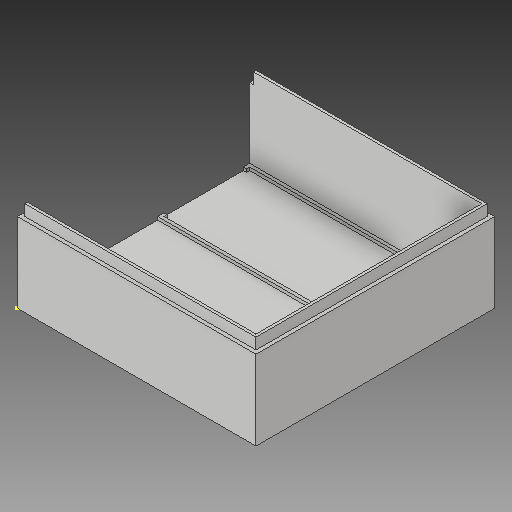
# Autodesk Inventor part: base inf
Saved by Autodesk Inventor 2018.2 (Build 222227000, 227)
## iProperties
Created: 2016-05-12
Part Number: base inf
Material: Genérico
Document SubType Name: Modeling
Designer: Usuario
Density: 1 g/cm^3
Appearance: Valor por defecto
Author: Usuario
Autodesk Inventor part; units mm, degrees
ref_plane "YZ Plane" through (0, 0, 0) normal (1, 0, 0) x (0, 1, 0)
ref_plane "XZ Plane" through (0, 0, 0) normal (0, 1, 0) x (-1, 0, 0)
ref_plane "XY Plane" through (0, 0, 0) normal (0, 0, 1) x (1, 0, 0)
sketch "Boceto1" plane through (0, 0, 0) normal (0, 1, 0) x (-1, 0, 0)
  line L0 (0, 0) -> (0, -150)
  line L1 (0, -150) -> (-150, -150)
  line L2 (-150, -150) -> (-150, 0)
  line L3 (-150, 0) -> (0, 0)
  constraints: 8 end point, 2 perpendicular, 1 vertical
extrude "Extrusión1" add sketch "Boceto1" along normal blind 4
sketch "Boceto2" plane through (0, 4, 0) normal (0, 1, 0) x (1, 0, 0)
  line L0 (0, 150) -> (4, 150)
  line L1 (150, 150) -> (0, 150) projected
  line L2 (0, 150) -> (0, 0)
  line L3 (0, 0) -> (150, 0)
  line L4 (150, 0) -> (150, 150)
  line L5 (0, 150) -> (150, 150)
  line L6 (4, 4) -> (146, 4)
  line L7 (146, 146) -> (146, 4)
  line L8 (146, 146) -> (4, 146)
  line L9 (4, 4) -> (4, 146)
  constraints: 18 end point, 4 perpendicular, 1 horizontal, 1 point on line, 1 vertical
extrude "Extrusión2" add sketch "Boceto2" along normal blind 46
sketch "Boceto3" plane through (0, 0, 0) normal (0, 0, 1) x (1, 0, 0)
  point P0 (0, 0)
sketch "Boceto4" plane through (0, 50, 0) normal (0, 1, 0) x (1, 0, 0)
  line L0 (4, 146) -> (146, 146) projected
  line L1 (0, 0) -> (0, 150) projected
  line L2 (146, 4) -> (4, 4) projected
  line L3 (2.3, 4) -> (2.3, 147.7)
  line L4 (2.3, 4) -> (2.3, 2.3)
  line L5 (2.3, 2.3) -> (147.7, 2.3)
  line L6 (147.7, 147.7) -> (2.3, 147.7)
  line L7 (147.7, 147.7) -> (147.7, 2.3)
  line L8 (4, 146) -> (146, 146)
  line L9 (146, 146) -> (146, 4) projected
  line L10 (146, 4) -> (146, 146)
  line L11 (4, 146) -> (4, 4)
  line L12 (4, 4) -> (146, 4)
  constraints: 18 end point, 5 perpendicular, 1 collinear, 1 parallel, 1 vertical
extrude "Extrusión3" add sketch "Boceto4" along normal blind 7
sketch "Boceto5" plane through (0, 0, -150) normal (-1, 0, 0) x (0, 0, 1)
  point P0 (150, 0)
sketch "Boceto6" plane through (0, 0, -150) normal (-1, 0, 0) x (0, 0, 1)
  line L0 (0, 0) -> (0, 50) projected
  line L1 (0, 50) -> (4, 50)
  line L2 (0, 50) -> (150, 50) projected
  line L3 (146, 4) -> (4, 4) projected
  line L4 (4, 4) -> (4, 50)
  line L5 (4, 4) -> (146, 4)
  line L6 (146, 4) -> (146, 57) projected
  line L7 (146, 4) -> (146, 50)
  line L8 (146, 50) -> (4, 50)
  line L9 (147.7, 50) -> (2.3, 50) projected
  point P0 (150, 0)
  constraints: 10 end point, 3 point on line, 2 collinear, 1 perpendicular
extrude "Extrusión4" cut sketch "Boceto6" against normal blind 4
sketch "Boceto7" plane through (2.3, 50, -2.3) normal (-1, 0, 0) x (0, 0, 1)
  line L0 (-1.7, -46) -> (-1.7, 7) projected
  line L1 (-1.7, 0) -> (-1.7, 7)
  line L2 (-143.7, -46) -> (-143.7, 7) projected
  line L3 (-1.7, 7) -> (-143.7, 7)
  line L4 (-143.7, 7) -> (-143.7, 0)
  line L5 (2.3, 0) -> (-147.7, 0) projected
  line L6 (-143.7, 0) -> (-1.7, 0)
  point P0 (2.3, -50)
  constraints: 8 end point, 2 perpendicular, 2 point on line, 1 collinear, 1 vertical
extrude "Extrusión5" cut sketch "Boceto7" against normal blind 4
sketch "Boceto8" plane through (0, 4, 0) normal (0, 1, 0) x (1, 0, 0)
  line L0 (0, 88.1) -> (106.1, 88.1)
  line L1 (106.1, 88.1) -> (106.1, 146)
  line L2 (0, 4) -> (0, 146) projected
  line L3 (0, 88.1) -> (0, 90.1)
  line L4 (2, 90.1) -> (104.1, 90.1)
  line L5 (106.1, 88.1) -> (104.1, 88.1)
  line L6 (104.1, 90.1) -> (104.1, 144)
  line L7 (106.1, 146) -> (106.1, 144)
  line L8 (104.1, 144) -> (2, 144)
  line L9 (0, 146) -> (106.1, 146)
  line L10 (2, 144) -> (2, 142)
  line L11 (2, 142) -> (0, 142)
  line L12 (2, 90.1) -> (2, 92.1)
  line L13 (2, 92.1) -> (0, 92.1)
  line L14 (0, 146) -> (0, 142)
  line L15 (0, 92.1) -> (0, 88.1)
  line L16 (2, 144) -> (2, 142)
  line L17 (2, 92.1) -> (2, 90.1)
  line L18 (0, 52) -> (48, 52)
  line L19 (48, 52) -> (48, 4)
  line L20 (0, 4) -> (146, 4) projected
  line L21 (2.3, 4) -> (0, 4) projected
  line L22 (0, 4) -> (48, 4)
  line L23 (2.3, 2.3) -> (147.7, 2.3) projected
  line L24 (0, 52) -> (0, 50)
  line L25 (2, 50) -> (46, 50)
  line L26 (46, 50) -> (46, 6)
  line L27 (46, 6) -> (2, 6)
  line L28 (0, 4) -> (48, 4)
  line L29 (0, 4) -> (48, 4)
  line L30 (2, 6) -> (2, 8)
  line L31 (2, 8) -> (0, 8)
  line L32 (2, 50) -> (2, 48)
  line L33 (2, 48) -> (0, 48)
  line L34 (2, 6) -> (2, 8)
  line L35 (2, 48) -> (2, 50)
  line L36 (0, 4) -> (0, 8)
  line L37 (0, 48) -> (0, 52)
  line L38 (0, 142) -> (0, 146)
  line L39 (0, 146) -> (106.1, 146)
  line L40 (2.3, 146) -> (146, 146) projected
  line L41 (106.1, 146) -> (106.1, 88.1)
  line L42 (106.1, 88.1) -> (0, 88.1)
  line L43 (0, 88.1) -> (0, 92.1)
  line L44 (0, 92.1) -> (2, 92.1)
  line L45 (2, 92.1) -> (2, 90.1)
  line L46 (2, 90.1) -> (104.1, 90.1)
  line L47 (104.1, 90.1) -> (104.1, 144)
  line L48 (104.1, 144) -> (2, 144)
  line L49 (2, 144) -> (2, 142)
  line L50 (2, 142) -> (0, 142)
  line L51 (0, 146) -> (2.3, 146) projected
  line L52 (0, 142) -> (0, 146)
  point P0 (0, 0)
  constraints: 94 end point, 22 perpendicular, 9 collinear, 7 point on line, 3 vertical, 1 horizontal, 1 midpoint, 1 parallel
extrude "Extrusión6" add sketch "Boceto8" along normal blind 2 contours L18 L19 L20 L2 L31 L30 L27 L26 L25 L32 L33
sketch "Boceto9" plane through (0, 4, 0) normal (0, 1, 0) x (1, 0, 0)
  line L0 (0, 88.1) -> (106.1, 88.1)
  line L1 (106.1, 88.1) -> (106.1, 146)
  line L2 (0, 88.1) -> (0, 90.1)
  line L3 (2, 90.1) -> (104.1, 90.1)
  line L4 (106.1, 88.1) -> (104.1, 88.1)
  line L5 (104.1, 90.1) -> (104.1, 144)
  line L6 (106.1, 146) -> (106.1, 144)
  line L7 (104.1, 144) -> (2, 144)
  line L8 (0, 146) -> (106.1, 146)
  line L9 (2, 144) -> (2, 142)
  line L10 (2, 142) -> (0, 142)
  line L11 (2, 90.1) -> (2, 92.1)
  line L12 (2, 92.1) -> (0, 92.1)
  line L13 (0, 146) -> (0, 142)
  line L14 (0, 92.1) -> (0, 88.1)
  line L15 (2, 144) -> (2, 142)
  line L16 (2, 92.1) -> (2, 90.1)
  line L17 (0, 142) -> (0, 146)
  line L18 (0, 146) -> (106.1, 146)
  line L19 (106.1, 146) -> (106.1, 88.1)
  line L20 (106.1, 88.1) -> (0, 88.1)
  line L21 (0, 88.1) -> (0, 92.1)
  line L22 (0, 92.1) -> (2, 92.1)
  line L23 (2, 92.1) -> (2, 90.1)
  line L24 (2, 90.1) -> (104.1, 90.1)
  line L25 (104.1, 90.1) -> (104.1, 144)
  line L26 (104.1, 144) -> (2, 144)
  line L27 (2, 144) -> (2, 142)
  line L28 (2, 142) -> (0, 142)
  line L29 (0, 146) -> (2.3, 146)
  line L30 (0, 142) -> (0, 146)
  point P0 (0, 0)
  point P1 (0, 52)
  constraints: 62 end point, 12 perpendicular, 5 collinear, 2 point on line, 2 vertical, 1 horizontal
extrude "Extrusión7" add sketch "Boceto9" along normal blind 2
